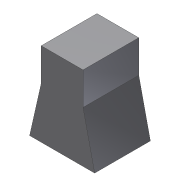
# Autodesk Inventor part: Conveyor_Representation_FloorPickup
Saved by Autodesk Inventor 2012 (Build 160160000, 160)
## iProperties
Created: 2012-01-09
Part Number: Conveyor_Representation_FloorPickup
Material: Default
Document SubType Name: Modeling
Designer: JesseK
Density: 1 g/cm^3
Mass: 24842.8 g
Surface Area: 5519.27 cm^2
Volume: 24842.8 cm^3
Author: JesseK
Autodesk Inventor part; units mm, degrees
ref_plane "YZ Plane" through (0, 0, 0) normal (1, 0, 0) x (0, 1, 0)
ref_plane "XZ Plane" through (0, 0, 0) normal (0, 1, 0) x (-1, 0, 0)
ref_plane "XY Plane" through (0, 0, 0) normal (0, 0, 1) x (1, 0, 0)
sketch "Sketch1" plane through (0, 0, 0) normal (0, 0, 1) x (1, 0, 0)
  line L0 (0, 0) -> (355.6, 0)
  line L1 (355.6, 0) -> (355.6, 457.2)
  line L2 (355.6, 457.2) -> (0, 457.2)
  line L3 (0, 457.2) -> (0, 0)
  dimension "d2" = 355.6
  dimension "d3" = 457.2
  constraints: 8 end point, 2 parallel, 1 horizontal, 1 perpendicular
  measures "d2" distance of L1.end L2.end
  measures "d3" distance of L2.end L0.start
extrude "Extrusion1" add sketch "Sketch1" along normal blind 203.2
sketch "Sketch2" plane through (0, 0, 203.2) normal (0, 0, 1) x (1, 0, 0)
  line L0 (0, 0) -> (0, 457.2) projected
  line L1 (355.6, 0) -> (0, 0) projected
  line L2 (355.6, 457.2) -> (355.6, 0) projected
  line L3 (0, 457.2) -> (355.6, 457.2) projected
  line L4 (0, 279.4) -> (63.5, 279.4) construction
  line L5 (63.5, 279.4) -> (292.1, 279.4) construction
  line L6 (292.1, 279.4) -> (355.6, 279.4) construction
  line L7 (63.5, 279.4) -> (0, 0)
  line L8 (292.1, 279.4) -> (355.6, 0)
  line L9 (63.5, 279.4) -> (63.5, 457.2)
  line L10 (0, 457.2) -> (0, 0)
  line L11 (292.1, 279.4) -> (292.1, 457.2)
  line L12 (355.6, 457.2) -> (355.6, 0)
  dimension "d4" = 279.4
  dimension "d5" = 228.6
  constraints: 18 end point, 4 point on line, 3 collinear, 3 perpendicular, 2 parallel
  measures "d4" distance between parallel lines of L1 L5
  measures "d5" distance of L4.end L5.end
extrude "Extrusion2" cut sketch "Sketch2" against normal up to next contours L0 L3 L9 L7 | L8 L11 L3 L2
body "Solid1"
